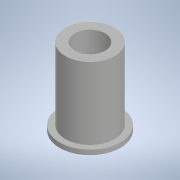
# Autodesk Inventor part: Barrel End Cap
Saved by Autodesk Inventor 2020 (Build 240168000, 168)
## iProperties
Created: 2020-03-16
Part Number: Barrel End Cap
Material: Generic
Document SubType Name: Modeling
Designer: Daniel
Density: 1 g/cm^3
Appearance: Light Gray
Author: Daniel
Autodesk Inventor part; units mm, degrees
ref_plane "YZ Plane" through (0, 0, 0) normal (1, 0, 0) x (0, 1, 0)
ref_plane "XZ Plane" through (0, 0, 0) normal (0, 1, 0) x (-1, 0, 0)
ref_plane "XY Plane" through (0, 0, 0) normal (0, 0, 1) x (1, 0, 0)
sketch "Sketch1" plane through (0, 0, 0) normal (0, 0, 1) x (1, 0, 0)
  line L0 (0, 0) -> (3.302, 0)
  line L1 (3.302, 0) -> (3.302, 9.652)
  line L2 (2.032, 9.652) -> (3.302, 9.652)
  line L3 (3.302, 9.652) -> (3.302, 0)
  line L4 (3.302, 0) -> (2.032, 0)
  line L5 (2.032, 0) -> (2.032, 9.652)
  line L6 (0, 9.652) -> (0, 0)
  line L7 (0, 0) -> (4.0831, 0)
  line L8 (0, -1.524) -> (0, 0)
  line L9 (4.0831, -0.635) -> (2.2225, -1.524)
  line L10 (0, -1.524) -> (2.2225, -1.524)
  line L11 (3.302, 0) -> (4.0831, 0)
  line L12 (4.0831, -0.635) -> (4.0831, 0)
  dimension "d0" = 9.652
  dimension "d3" = 1.27
  dimension "d4" = 3.302
  dimension "d7" = 0.635
  dimension "d8" = 2.2225
  constraints: 26 end point, 4 horizontal, 3 perpendicular, 2 parallel, 1 collinear, 1 vertical
  measures "d0" distance of L0.end L1.end
  measures "d3" distance of L2.start L2.end
  measures "d4" distance between parallel lines of L1 L6
  measures "d7" distance of L7.end L9.start
  measures "d8" distance of L9.end L8.start
revolve "Revolution1" add sketch "Sketch1" angle 360 about axis through (0, 9.652, 0) along (0, -1, 0)
body "Solid1"
